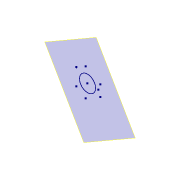
# Autodesk Inventor part: 20_Cube_Insert_Openflexure_Deltastage_Adapter
Saved by Autodesk Inventor 2019.4 (Build 234330000, 330)
## iProperties
Created: 2019-11-15
Part Number: 20_Cube_Insert_Openflexure_Deltastage_Adapter
Material: Generic
Document SubType Name: Modeling
Designer: diederichbenedict
Density: 1 g/cm^3
Appearance: Default
Author: diederichbenedict
Autodesk Inventor part; units mm, degrees
ref_plane "YZ Plane" through (0, 0, 0) normal (1, 0, 0) x (0, 1, 0)
ref_plane "XZ Plane" through (0, 0, 0) normal (0, 1, 0) x (-1, 0, 0)
ref_plane "XY Plane" through (0, 0, 0) normal (0, 0, 1) x (1, 0, 0)
ref_plane "Work Plane4" through (23.7495, -12.4998, 8) normal (0, 0, -1) x (0.866, 0.5, 0)
sketch "Sketch9" plane through (23.7495, -12.4998, 8) normal (0, 0, -1) x (0.866, 0.5, 0)
  circle A0 centre (-36.9735, 7.7008) radius 1.3002
  circle A1 centre (8.3375, 7.7008) radius 1.3002
  circle A2 centre (23.3378, -18.28) radius 1.3
  circle A3 centre (-14.318, -22.6998) radius 21.9102
  circle A4 centre (-51.9737, -18.28) radius 1.3001
  line L0 (-27.63, -57.387) -> (-29.04, -59.377)
  circle A5 centre (-29.3181, -57.5206) radius 1.3001
  circle A6 centre (0.6822, -57.5205) radius 1.3
  circle A7 centre (11.5075, -7.7902) radius 1.3002
  line L1 (-33.586, -63.403) -> (4.877, -63.403) construction
  line L2 (-39.9342, 14.3381) -> (-59.166, -18.972) construction
  line L3 (30.566, -19.035) -> (11.3349, 14.275) construction
  line L4 (-14.3189, -92.6998) -> (-74.9393, 12.301) construction
  line L5 (-74.9393, 12.301) -> (46.3042, 12.2995) construction
  line L6 (46.3042, 12.2995) -> (-14.3189, -92.6998) construction
  line L7 (41.198, -34.545) -> (23.698, -64.855) construction
  line L8 (2.5961, -63.403) -> (-31.2329, -63.403)
  line L9 (-31.2329, -63.403) -> (-58.0252, -16.9961)
  line L10 (-58.0252, -16.9961) -> (-41.1106, 12.3006)
  line L11 (-41.1106, 12.3006) -> (12.4752, 12.2999)
  line L12 (12.4752, 12.2999) -> (29.3894, -16.997)
  line L13 (29.3894, -16.997) -> (2.5961, -63.403)
  point P0 (-14.318, -22.6998)
  dimension "d56" = 35
  constraints: 28 end point, 12 point on line, 8 centre point, 1 coincident, 1 horizontal, 1 parallel, 37 other
  measures "d56" distance from line of point (-14.318, -22.7) L6
extrude "Extrusion4" add sketch "Sketch9" along normal blind 3
sketch "Sketch10" plane through (23.7495, -12.4998, 5) normal (0, 0, -1) x (-0.866, -0.5, 0)
  circle A0 centre (14.318, 22.6998) radius 21.9102 projected
  circle A1 centre (36.9735, -7.7008) radius 1.3002 projected
  circle A2 centre (-8.3375, -7.7008) radius 1.3002 projected
  circle A3 centre (-11.5075, 7.7902) radius 1.3002 projected
  circle A4 centre (29.3181, 57.5206) radius 1.3001 projected
  circle A5 centre (51.9737, 18.28) radius 1.3001 projected
  circle A6 centre (-23.3378, 18.28) radius 1.3 projected
  circle A7 centre (-0.6822, 57.5205) radius 1.3 projected
  line L0 (31.2329, 63.403) -> (-2.5961, 63.403) projected
  line L1 (-2.5961, 63.403) -> (-29.3894, 16.997) projected
  line L2 (-29.3894, 16.997) -> (-12.4752, -12.2999) projected
  line L3 (-12.4752, -12.2999) -> (41.1106, -12.3006) projected
  line L4 (41.1106, -12.3006) -> (58.0252, 16.9961) projected
  line L5 (58.0252, 16.9961) -> (31.2329, 63.403) projected
  line L6 (32.318, -14.6138) -> (-3.682, -14.6138)
  line L7 (-3.682, -14.6138) -> (-3.682, -4.5139)
  line L8 (-3.682, -4.5139) -> (32.318, -4.5139)
  line L9 (32.318, -4.5139) -> (32.318, -14.6138)
  point P0 (14.318, 22.6998)
  dimension "d59" = 18
  dimension "d60" = 18
  constraints: 8 end point, 2 parallel, 1 horizontal, 1 perpendicular
  measures "d59" distance from line of L7 point (14.318, 22.7)
  measures "d60" distance from line of point (14.318, 22.7) L9
extrude "Extrusion5" cut sketch "Sketch10" against normal through all contours L9 L6 L7 L3 | L3 L7 L8 L9
pattern_circular "Circular Pattern1" count 3 over 360 about axis through (0, 0, 8) along (0, 0, -1) of "Extrusion5"
sketch "Sketch11" plane through (23.7495, -12.4998, 5) normal (0, 0, -1) x (-0.866, -0.5, 0)
  line L0 (23.469, 56.8503) -> (-7.8173, 38.7876)
  line L1 (-15.8275, 24.9136) -> (5.167, -11.4508)
  line L2 (5.167, -11.4508) -> (48.4685, 13.5488)
  line L3 (48.4685, 13.5488) -> (23.469, 56.8503)
  line L4 (23.469, 56.8503) -> (5.167, -11.4508) construction
  line L5 (-19.8325, 31.8507) -> (48.4685, 13.5488) construction
  line L6 (-2.59, 41.8055) -> (-7.8173, 38.7876)
  circle A0 centre (14.318, 22.6998) radius 21.9102 projected
  line L7 (-0.2497, 51.8951) -> (-18.2497, 20.7181) projected
  line L8 (-3.682, -4.5139) -> (32.318, -4.5139) projected
  point P0 (14.318, 22.6998)
  point P1 (1.1621, -4.5139)
  point P2 (17.1824, -4.5139)
  dimension "d66" = 50
  dimension "d67" = 50
  constraints: 14 end point, 6 point on line, 2 midpoint, 2 parallel, 1 collinear, 1 perpendicular, 3 other
  measures "d66" distance of L0.start L5.start
  measures "d67" distance of L1.end L5.start
extrude "Extrusion6" add sketch "Sketch11" along normal blind 3 contours L3 L2 L8 L1 L7 L0
sketch "Sketch12" plane through (23.7495, -12.4998, 2) normal (0, 0, -1) x (-0.866, -0.5, 0)
  circle A0 centre (37.2753, 11.9362) radius 2.65
  circle A1 centre (39.5813, 20.5422) radius 2.65
  circle A2 centre (25.0816, 45.657) radius 2.65
  circle A3 centre (16.4756, 47.9631) radius 2.65
  circle A4 centre (-10.9453, 24.8574) radius 2.65
  circle A5 centre (3.5544, -0.2575) radius 2.65
  circle A6 centre (12.1604, -2.5635) radius 2.65
  circle A7 centre (-8.6393, 33.4633) radius 2.65
  point P0 (14.318, 22.6998)
  constraints: 8 centre point, 1 coincident, 16 other
hole "Hole4" at (-20.8, -14.5, 2) at (-14.5, -20.8, 2) at (20.8, -14.5, 2) at (20.8, 14.5, 2) at (-14.5, 20.8, 2) at (-20.8, 14.5, 2) direction (0, 0, 1) diameter 4.8 end through all
body "Solid2"
